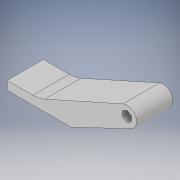
# Autodesk Inventor part: Brace
Saved by Autodesk Inventor 2019.4 (Build 234330000, 330)
## iProperties
Created: 2020-04-17
Part Number: Brace
Material: Generic
Document SubType Name: Modeling
Designer: admin
Density: 1 g/cm^3
Appearance: Default
Author: admin
Autodesk Inventor part; units mm, degrees
ref_plane "YZ Plane" through (0, 0, 0) normal (1, 0, 0) x (0, 1, 0)
ref_plane "XZ Plane" through (0, 0, 0) normal (0, 1, 0) x (-1, 0, 0)
ref_plane "XY Plane" through (0, 0, 0) normal (0, 0, 1) x (1, 0, 0)
sketch "Sketch1" plane through (0, 0, 0) normal (0, 0, 1) x (1, 0, 0)
  line L0 (0, 0) -> (88.085, 0) construction
  circle A0 centre (0, 0) radius 22.25 construction
  line L1 (92.335, -2.4537) -> (88.085, -4.9075)
  line L2 (88.085, -4.9075) -> (83.835, -2.4537)
  line L3 (83.835, -2.4537) -> (83.835, 2.4537)
  line L4 (83.835, 2.4537) -> (88.085, 4.9075)
  line L5 (88.085, 4.9075) -> (92.335, 2.4537)
  line L6 (92.335, 2.4537) -> (92.335, -2.4537)
  line L7 (-24.1413, -35) -> (35.8587, -35)
  line L8 (-24.1413, -35) -> (-24.1413, -27)
  line L9 (-24.1413, -27) -> (0, -27)
  arc A1 (0, -27) -> (11.0348, -24.6421) centre (0, 0) ccw
  circle A2 centre (88.085, 0) radius 9
  line L10 (35.8587, -35) -> (91.9735, -8.1166)
  line L11 (11.0348, -24.6421) -> (84.4067, 8.214)
  point P0 (92.335, 0)
  dimension "d0" = 88.085
  dimension "d1" = 44.5
  dimension "d2" = 8.5
  dimension "d12" = 35
  dimension "d13" = 18
  dimension "d14" = 8
  dimension "d15" = 60
  constraints: 24 end point, 4 coincident, 4 point on circle, 4 tangent, 3 centre point, 2 horizontal, 1 midpoint, 1 perpendicular, 1 point on line, 1 vertical, 13 other
  measures "d0" distance of L0.start L0.end
  measures "d1" diameter of A0
  measures "d2" distance between parallel lines of L3 L6
  measures "d12" distance from line of A0.centre L7
  measures "d13" diameter of A2
  measures "d14" distance of L7.start L8.end
  measures "d15" distance of L7.start L7.end
extrude "Extrusion1" add sketch "Sketch1" along normal mid plane 34
sketch "Sketch2" plane through (0, 0, 17) normal (0, 0, 1) x (1, 0, 0)
  line L0 (88.085, -4.9075) -> (83.835, -2.4537) projected
  line L1 (83.835, -2.4537) -> (83.835, 2.4537) projected
  line L2 (83.835, 2.4537) -> (88.085, 4.9075) projected
  line L3 (88.085, 4.9075) -> (92.335, 2.4537) projected
  line L4 (92.335, 2.4537) -> (92.335, -2.4537) projected
  line L5 (92.335, -2.4537) -> (88.085, -4.9075) projected
  line L6 (3.9734, 19.6013) -> (27.3169, 14.8693) construction
  arc A0 (88.5817, -2.4502) -> (88.5817, 2.4502) centre (88.085, 0) ccw construction
  line L7 (88.5817, -2.4502) -> (74.6189, -5.2806) construction
  arc A1 (3.9734, 19.6013) -> (3.9734, -19.6013) centre (0, 0) ccw construction
  line L8 (74.6189, 5.2806) -> (74.6189, -5.2806)
  line L9 (27.3169, 14.8693) -> (27.3169, -14.8693)
  line L10 (30.5542, 14.2131) -> (50.2765, -10.2151)
  line L11 (38.3021, 12.6425) -> (55.8449, -9.0863)
  line L12 (38.3021, 12.6425) -> (74.6189, 5.2806)
  line L13 (74.6189, 5.2806) -> (88.5817, 2.4502) construction
  line L14 (27.3169, 14.8693) -> (30.5542, 14.2131)
  line L15 (30.5542, 14.2131) -> (38.3021, 12.6425) construction
  line L16 (50.2765, -10.2151) -> (27.3169, -14.8693)
  line L17 (27.3169, -14.8693) -> (3.9734, -19.6013) construction
  line L18 (74.6189, -5.2806) -> (55.8449, -9.0863)
  line L19 (55.8449, -9.0863) -> (50.2765, -10.2151) construction
  constraints: 28 end point, 4 point on circle, 4 point on line, 2 centre point, 2 parallel, 1 vertical
extrude "Extrusion2" [suppressed]
fillet "Fillet1" [suppressed]
fillet "Fillet2" [suppressed]
body "Solid1"
